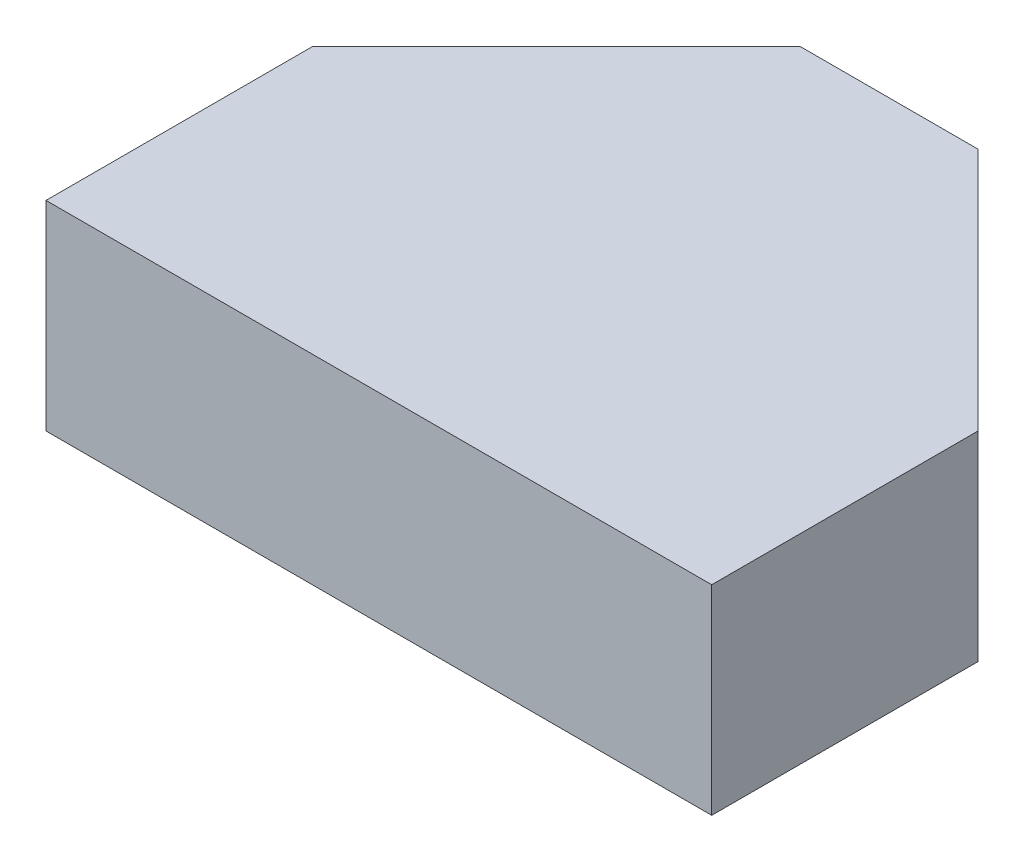
# Autodesk Inventor part: DUMMY 2
Saved by Autodesk Inventor 2024.2 (Build 282272000, 272)
## iProperties
Created: 2024-06-16
Part Number: DUMMY 2
Material: Generic
Document SubType Name: Modeling
Designer: admin
Mass: 640125 g
Surface Area: 49400.4 cm^2
Volume: 640125 cm^3
Density: 1 g/cm^3
Appearance: Default
Author: admin
Autodesk Inventor part; units mm, degrees
ref_plane "YZ Plane" through (0, 0, 0) normal (1, 0, 0) x (0, 1, 0)
ref_plane "XZ Plane" through (0, 0, 0) normal (0, 1, 0) x (-1, 0, 0)
ref_plane "XY Plane" through (0, 0, 0) normal (0, 0, 1) x (1, 0, 0)
sketch "Sketch1" plane through (0, 0, 0) normal (0, 1, 0) x (-1, 0, 0)
  line L0 (200, 0) -> (-200, 0)
  line L1 (200, 0) -> (750, 550)
  line L2 (750, 550) -> (750, 1150)
  line L3 (750, 1150) -> (-750, 1150)
  line L4 (-750, 1150) -> (-750, 550)
  line L5 (-750, 550) -> (-200, 0)
  point P0 (0, 0)
  point P1 (0, 0)
  point P2 (0, 1150)
  dimension "d0" = 400
  dimension "d1" = 1150
  dimension "d2" = 600
  dimension "d3" = 1500
  constraints: 12 end point, 3 perpendicular, 2 midpoint, 1 coincident, 1 horizontal, 1 horizontal alignment, 1 vertical, 1 vertical alignment
  measures "d0" distance of L0.start L0.end
  measures "d1" distance between parallel lines of L0 L3
  measures "d2" distance of L1.end L2.end
  measures "d3" distance of L2.end L3.end
extrude "Extrusion1" add sketch "Sketch1" along normal blind 450
body "Solid1"
